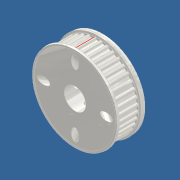
# Autodesk Inventor part: 10-03-035 roata condusa GT2
Saved by Autodesk Inventor 2020 (Build 240168000, 168)
## iProperties
CustomPartVersion: 1
Created: 2020-05-09
Part Number: 10-03-035 roata condusa GT2
Material: Steel
Document SubType Name: Modeling
Designer: 40743
Density: 7.85 g/cm^3
Appearance: Steel
Description: Roata GT2
Mass: 70.7378 g
Surface Area: 45.9795 cm^2
Volume: 9.01118 cm^3
Author: 40743
Subject: 015
Autodesk Inventor part; units mm, degrees
ref_plane "YZ Plane" through (0, 0, 0) normal (1, 0, 0) x (0, 1, 0)
ref_plane "XZ Plane" through (0, 0, 0) normal (0, 1, 0) x (-1, 0, 0)
ref_plane "XY Plane" through (0, 0, 0) normal (0, 0, 1) x (1, 0, 0)
sketch "Pulley Sketch" plane through (0, 0, 0) normal (0, 0, 1) x (1, 0, 0)
  circle A0 centre (0, 0) radius 15.9155 construction
  circle A1 centre (0, 0) radius 15.6155
  circle A2 centre (0, 0) radius 14.8655
  line L0 (-0.8636, 15.5916) -> (-0.525, 14.8655)
  line L1 (-0.525, 14.8655) -> (0.525, 14.8655)
  line L2 (0.525, 14.8655) -> (0.8636, 15.5916)
  line L3 (0, 0) -> (0, 15.6155) construction
  point P0 (0, 14.8655)
  dimension "d0" = 31.831
  dimension "d1" = 0.3
  dimension "d2" = 0.75
  dimension "d3" = 50
  dimension "d4" = 1.05
  constraints: 8 end point, 3 coincident, 3 point on circle, 2 centre point, 1 horizontal, 1 midpoint, 1 point on line, 1 vertical, 1 vertical alignment, 3 other
  measures "d0" diameter of A0
  measures "d1" radial gap between concentric circles of A0 A1
  measures "d3" angle of L2 L0
  measures "d4" distance of L0.end L1.end
extrude "Base Body" add sketch "Pulley Sketch" along normal mid plane 8 contours A2 | A1 L0 L1 L2 | L2 L1 L0 A1
extrude "Tooth" cut sketch "Pulley Sketch" along normal through all both and the other way through all contours L2 L1 L0 A1 picked at (0, 15.3637)
fillet "Tooth Fillet" radius 0.2 2 edges at (0.525, 14.8655, 0) (-0.525, 14.8655, 0)
fillet "Tooth Fillet" radius 0.3 4 edges at (-0.8636, 15.5916, 2) (-0.8636, 15.5916, -2) (0.8636, 15.5916, 2) (0.8636, 15.5916, -2)
pattern_circular "Teeth" count 40 over 360 about axis through (0, 0, -10) along (0, 0, 1) of "Tooth", "Tooth Fillet"
pulley flange "Left flange" diameter 31.231 height 0.8 thickness 0.8 bend angle 10 centre (0, 0, -4) toward (0, 0, -1)
pulley flange "Right flange" diameter 31.231 height 0.8 thickness 0.8 bend angle 10 centre (0, 0, 4) toward (0, 0, 1)
sketch "Sketch2" plane through (0, 0, -4.8) normal (0, 0, -1) x (-1, 0, 0)
  point P0 (0, 0)
  point P1 (0, 0)
  constraints: 1 coincident
hole "Hole1" at (0, 0, -4.8) direction (0, 0, 1) diameter 8.3 end through all
sketch "Sketch3" plane through (0, 0, -4.8) normal (0, 0, -1) x (-1, 0, 0)
  circle A0 centre (0, 0) radius 4.2 projected
  circle A1 centre (0, 0) radius 5.5
  point P0 (0, 0)
  dimension "d24" = 11
  constraints: 1 centre point, 1 coincident
  measures "d24" diameter of A1
extrude "Extrusion3" add sketch "Sketch3" along normal blind 2
ref_plane "Work Plane3" through (1.8222, 14.5772, 4.55) normal (0, 0.819152, 0.5735764) x (-1, 0, 0)
sketch "Sketch9" plane through (1.8222, 14.5772, 4.55) normal (0, 0.819152, 0.5735764) x (-1, 0, 0)
  point P0 (1.8222, 4.634)
  point P1 (1.8222, 1.634)
  dimension "d32" = 3
  constraints: 1 vertical alignment
  measures "d32" distance of point (1.822, 1.634) point (1.822, 4.634)
hole "Hole2" at (0, 13.64, 5.8885) direction (0, -0.819152, -0.5735764) diameter 2.8 depth 15
pattern_circular "Circular Pattern2" count 4 over 360 about axis through (0, 0, 4.5226) along (0, 0, 1) of "Hole2"
sketch "Sketch10" plane through (0, 0, -4.8) normal (0, 0, -1) x (-1, 0, 0)
  circle A0 centre (0, 0) radius 5.5 projected
  circle A1 centre (0, 0) radius 4.2 projected
  circle A2 centre (0, 0) radius 16.2766 projected
  point P0 (0, 0)
extrude "Extrusion5" add sketch "Sketch10" along normal blind 1 contours A2
equation "\"d1\" = da_a"
equation "\"d2\" = da_hg"
equation "\"d3\" = 2 * da_fi"
equation "\"d4\" = da_bw"
equation "\"d5\" = da_bf"
equation "\"d7\" = da_bf"
equation "\"d9\" = da_rb"
equation "\"d10\" = da_rt"
equation "\"da_pb\" = 2.5"
equation "\"da_fi\" = 25deg"
equation "\"da_hg\" = 0.75"
equation "\"da_bw\" = 1.05"
equation "\"da_rb\" = 0.2"
equation "\"da_rt\" = 0.3"
equation "\"da_a\" = 0.3"
equation "\"da_bf\" = 8"
equation "\"da_wf\" = 0.8"
equation "\"da_hf\" = 0.8"
body "Solid1"
